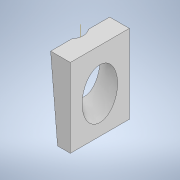
# Autodesk Inventor part: waterHeaterVent-V01
Saved by Autodesk Inventor 2021.1 (Build 251245010, 245A)
## iProperties
Created: 2020-10-25
Part Number: waterHeaterVent-V01
Material: Generic
Document SubType Name: Modeling
Designer: robst
Density: 1 g/cm^3
Appearance: Default
Author: robst
Autodesk Inventor part; units mm, degrees
ref_plane "YZ Plane" through (0, 0, 0) normal (1, 0, 0) x (0, 1, 0)
ref_plane "XZ Plane" through (0, 0, 0) normal (0, 1, 0) x (-1, 0, 0)
sketch "Sketch1" plane through (0, 0, 0) normal (0, 0, 1) x (1, 0, 0)
  line L0 (0, 0) -> (4.4444, -50.8)
  line L1 (0, -76.2) -> (0, 12.7) projected
  line L2 (0, 0) -> (12.7, 0)
  line L3 (12.7, 0) -> (12.7, -50.8)
  line L4 (4.4444, -50.8) -> (12.7, -50.8)
  dimension "d0" = 5
  dimension "d1" = 12.7
  dimension "d3" = 50.8
  constraints: 8 end point, 2 horizontal, 1 vertical
  measures "d0" angle of L0 L1
  measures "d1" distance of L0.start L2.end
  measures "d3" distance of L2.end L3.end
extrude "Extrusion1" add sketch "Sketch1" along normal mid plane 38.1
ref_plane "Work Plane1" through (12.7, -50.8, 0) normal (0.7071, -0.7071, 0) x (0, 0, 1)
sketch "Sketch2" plane through (12.7, -50.8, 0) normal (0.7071, -0.7071, 0) x (0, 0, 1)
  line L0 (19.05, 0) -> (19.05, -35.921) projected
  line L1 (19.05, -35.921) -> (-19.05, -35.921) projected
  line L2 (-19.05, -35.921) -> (-19.05, 0) projected
  line L3 (-19.05, 0) -> (19.05, 0) projected
  circle A0 centre (0, -16.871) radius 11.43
  point P0 (0, -26.9408)
  dimension "d7" = 22.86
  dimension "d10" = 19.05
  constraints: 1 centre point
  measures "d7" diameter of A0
  measures "d10" distance from line of A0.centre L1
extrude "Extrusion2" cut sketch "Sketch2" against normal through all contours A0
sketch "Sketch3" plane through (4.4444, -50.8, -19.05) normal (-0.9962, -0.0872, 0) x (0, 0, 1)
  line L0 (0, 0) -> (0, 50.994) construction
  line L1 (0, 10.16) -> (38.1, 10.16) construction
  line L2 (38.1, 50.994) -> (38.1, 0) construction
  line L3 (0, 0) -> (38.1, 0) construction
  line L4 (13.1178, 15.24) -> (9.6187, 5.08)
  line L5 (9.6187, 5.08) -> (8.1613, 5.08)
  line L6 (8.1613, 5.08) -> (4.6622, 15.24)
  line L7 (4.6622, 15.24) -> (6.1112, 15.24)
  line L8 (6.1112, 15.24) -> (8.9271, 6.8008)
  line L9 (8.9271, 6.8008) -> (11.7429, 15.24)
  line L10 (11.7429, 15.24) -> (13.1178, 15.24)
  line L11 (17.638, 8.9085) -> (13.793, 8.9085)
  line L12 (13.793, 8.9085) -> (13.793, 10.1435)
  line L13 (13.793, 10.1435) -> (17.638, 10.1435)
  line L14 (17.638, 10.1435) -> (17.638, 8.9085)
  spline S0 degree 2 poles (25.3115, 10.16) (25.3115, 7.4265) (23.7224, 4.8659) (22.0675, 4.8659) knots 0 0 0 1 2 2 2
  spline S1 degree 2 poles (22.0675, 4.8659) (20.3879, 4.8659) (18.8153, 7.4759) (18.8153, 10.1518) knots 0 0 0 1 2 2 2
  spline S2 degree 2 poles (18.8153, 10.1518) (18.8153, 12.9017) (20.4044, 15.4458) (22.0675, 15.4458) knots 0 0 0 1 2 2 2
  spline S3 degree 2 poles (22.0675, 15.4458) (23.7389, 15.4458) (25.3115, 12.8112) (25.3115, 10.16) knots 0 0 0 1 2 2 2
  spline S4 degree 2 poles (23.566, 7.0642) (23.7636, 7.5665) (23.9283, 9.1144) (23.9283, 10.16) knots 0 0 0 1 2 2 2
  spline S5 degree 2 poles (23.9283, 10.16) (23.9283, 11.2056) (23.7636, 12.7453) (23.5578, 13.264) knots 0 0 0 1 2 2 2
  spline S6 degree 2 poles (23.5578, 13.264) (23.3519, 13.7827) (22.6356, 14.3179) (22.0675, 14.3179) knots 0 0 0 1 2 2 2
  spline S7 degree 2 poles (22.0675, 14.3179) (21.4994, 14.3179) (20.7667, 13.7827) (20.5526, 13.2475) knots 0 0 0 1 2 2 2
  spline S8 degree 2 poles (20.5526, 13.2475) (20.3468, 12.7288) (20.1986, 11.148) (20.1986, 10.1518) knots 0 0 0 1 2 2 2
  spline S9 degree 2 poles (20.1986, 10.1518) (20.1986, 9.0814) (20.3303, 7.6488) (20.5444, 7.0889) knots 0 0 0 1 2 2 2
  spline S10 degree 2 poles (20.5444, 7.0889) (20.742, 6.562) (21.4747, 5.9939) (22.0675, 5.9939) knots 0 0 0 1 2 2 2
  spline S11 degree 2 poles (22.0675, 5.9939) (22.6274, 5.9939) (23.3602, 6.5291) (23.566, 7.0642) knots 0 0 0 1 2 2 2
  line L15 (32.3675, 5.08) -> (27.411, 5.08)
  line L16 (27.411, 5.08) -> (27.411, 6.1174)
  line L17 (27.411, 6.1174) -> (29.2553, 6.1174)
  line L18 (29.2553, 6.1174) -> (29.2553, 12.9264)
  line L19 (29.2553, 12.9264) -> (27.411, 12.9264)
  line L20 (27.411, 12.9264) -> (27.411, 13.8568)
  spline S12 degree 2 poles (27.411, 13.8568) (28.4566, 13.8568) (29.4447, 14.4496) (29.5105, 15.2729) knots 0 0 0 1 2 2 2
  line L21 (29.5105, 15.2729) -> (30.5644, 15.2729)
  line L22 (30.5644, 15.2729) -> (30.5644, 6.1174)
  line L23 (30.5644, 6.1174) -> (32.3675, 6.1174)
  line L24 (32.3675, 6.1174) -> (32.3675, 5.08)
  point P0 (19.05, 50.994)
  dimension "d12" = 10.16
  constraints: 2 end point, 2 horizontal, 2 point on line
  measures "d12" distance between parallel lines of L3 L1
extrude "Extrusion3" cut sketch "Sketch3" against normal blind 1.27
equation "\"d0\" = backAngle"
equation "\"d1\" = topPartDepth"
equation "\"d3\" = partHeight"
equation "\"d4\" = partWidth"
equation "\"d7\" = pipeExteriorDiameter"
equation "\"d10\" = pipeCenter"
equation "\"d13\" = textDepth"
equation "\"topPartDepth\" = 12.7"
equation "\"backAngle\" = 5deg"
equation "\"partHeight\" = 50.8"
equation "\"partWidth\" = 38.1"
equation "\"pipeExteriorDiameter\" = 22.86"
equation "\"pipeCenter\" = 19.05"
equation "\"filletEdge\" = 1.05833"
equation "\"textDepth\" = 1.27"
body "Solid1"
